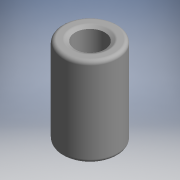
# Autodesk Inventor part: Part1
Saved by Autodesk Inventor 2016 (Build 200138000, 138)
## iProperties
Created: 2018-01-19
Part Number: Part1
Material: Generic
Document SubType Name: Modeling
Designer: student
Density: 1 g/cm^3
Appearance: Default
Author: student
Autodesk Inventor part; units mm, degrees
ref_plane "YZ Plane" through (0, 0, 0) normal (1, 0, 0) x (0, 1, 0)
ref_plane "XZ Plane" through (0, 0, 0) normal (0, 1, 0) x (-1, 0, 0)
ref_plane "XY Plane" through (0, 0, 0) normal (0, 0, 1) x (1, 0, 0)
sketch "Sketch1" plane through (0, 0, 0) normal (0, 1, 0) x (-1, 0, 0)
  circle A0 centre (12.2927, 22.2918) radius 4
  circle A1 centre (12.2927, 22.2918) radius 7.5
  point P0 (0, 0)
  dimension "d0" = 8
  dimension "d1" = 15
  constraints: 2 centre point, 1 coincident
  measures "d0" diameter of A0
  measures "d1" diameter of A1
extrude "Extrusion1" add sketch "Sketch1" along normal blind 24
chamfer "Chamfer1" distance 1 distance2 0.5 1 edges at (-8.2927, 24, 22.2918) measured on face at (-18.5146, 24, 21.3744)
fillet "Fillet2" radius 1 1 edges at (-4.7927, 24, 22.2918)
fillet "Fillet3" radius 1 1 edges at (-7.2927, 24, 22.2918)
chamfer "Chamfer2" distance 1 distance2 0.5 1 edges at (-8.2927, 0, 22.2918) measured on face at (-16.2409, 15.6667, 21.6501)
fillet "Fillet4" radius 1 1 edges at (-7.7927, 0, 22.2918)
fillet "Fillet5" radius 1 1 edges at (-4.7927, 0, 22.2918)
body "Solid1"
